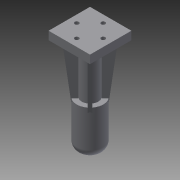
# Autodesk Inventor part: QuadrupedFoot
Saved by Autodesk Inventor 2015 (Build 190159000, 159)
## iProperties
Created: 2015-04-28
Part Number: QuadrupedFoot
Material: ABS Plastic
Document SubType Name: Modeling
Designer: Quinn
Density: 1.06 g/cm^3
Appearance: Smooth - White
Author: Quinn
Autodesk Inventor part; units mm, degrees
ref_plane "YZ Plane" through (0, 0, 0) normal (1, 0, 0) x (0, 1, 0)
ref_plane "XZ Plane" through (0, 0, 0) normal (0, 1, 0) x (-1, 0, 0)
ref_plane "XY Plane" through (0, 0, 0) normal (0, 0, 1) x (1, 0, 0)
sketch "Sketch2" plane through (0, 0, 0) normal (0, 1, 0) x (-1, 0, 0)
  line L0 (3.9404, 4.971) -> (-21.0596, 4.971)
  line L1 (-21.0596, 4.971) -> (-21.0596, -20.029)
  line L2 (-21.0596, -20.029) -> (3.9404, -20.029)
  line L3 (3.9404, -20.029) -> (3.9404, 4.971)
  circle A0 centre (-0.5596, -7.529) radius 1.25
  circle A1 centre (-16.5596, -7.529) radius 1.25
  circle A2 centre (-8.5596, 0.471) radius 1.25
  circle A3 centre (-8.5596, -15.529) radius 1.25
  point P0 (0, 0)
  dimension "d0" = 25
  dimension "d1" = 25
  dimension "d4" = 2.5
  dimension "d5" = 2.5
  dimension "d8" = 2.5
  dimension "d9" = 2.5
  constraints: 8 end point, 4 centre point, 2 parallel, 1 horizontal, 1 perpendicular
  measures "d0" distance of L2.end L1.end
  measures "d1" distance of L1.end L0.end
  measures "d4" diameter of A0
  measures "d5" diameter of A1
  measures "d8" diameter of A2
  measures "d9" diameter of A3
extrude "Extrusion1" add sketch "Sketch2" along normal blind 7
sketch "Sketch3" plane through (0, 0, 0) normal (0, -1, 0) x (1, 0, 0)
  circle A0 centre (8.5596, -15.529) radius 1.25 projected
  circle A1 centre (8.5596, 0.471) radius 1.25 projected
  circle A2 centre (16.5596, -7.529) radius 1.25 projected
  circle A3 centre (0.5596, -7.529) radius 1.25 projected
  line L0 (-3.9404, 4.971) -> (21.0596, 4.971) projected
  line L1 (-3.9404, -20.029) -> (-3.9404, 4.971) projected
  line L2 (21.0596, -20.029) -> (-3.9404, -20.029) projected
  line L3 (21.0596, 4.971) -> (21.0596, -20.029) projected
  circle A4 centre (8.5596, -7.529) radius 5
  point P0 (0, 0)
  dimension "d12" = 10
  constraints: 1 centre point
  measures "d12" diameter of A4
extrude "Extrusion2" add sketch "Sketch3" along normal blind 55 contours A4
sketch "Sketch4" plane through (0, 0, 0) normal (0, -1, 0) x (1, 0, 0)
  circle A0 centre (8.5596, -7.529) radius 5 projected
  circle A1 centre (8.5596, -15.529) radius 1.25 projected
  circle A2 centre (8.5596, 0.471) radius 1.25 projected
  circle A3 centre (16.5596, -7.529) radius 1.25 projected
  circle A4 centre (0.5596, -7.529) radius 1.25 projected
  line L0 (-3.9404, 4.971) -> (21.0596, 4.971) projected
  line L1 (-3.9404, -20.029) -> (-3.9404, 4.971) projected
  line L2 (21.0596, -20.029) -> (-3.9404, -20.029) projected
  line L3 (21.0596, 4.971) -> (21.0596, -20.029) projected
  circle A5 centre (8.5596, -15.529) radius 2.25
  circle A6 centre (16.5596, -7.529) radius 2.25
  circle A7 centre (8.5596, 0.471) radius 2.25
  circle A8 centre (0.5596, -7.529) radius 2.25
  point P0 (0, 0)
  dimension "d15" = 1
  dimension "d16" = 1
  dimension "d17" = 1
  dimension "d18" = 1
  constraints: 4 centre point
  measures "d15" radial gap between concentric circles of A1 A5
  measures "d16" radial gap between concentric circles of A3 A6
  measures "d17" radial gap between concentric circles of A2 A7
  measures "d18" radial gap between concentric circles of A4 A8
extrude "Extrusion3" cut sketch "Sketch4" against normal blind 2 contours A5 | A6 | A7 | A8
ref_plane "Work Plane1" through (-3.9404, 0, -20.029) normal (-0.7071068, 0, 0.7071068) x (0, 1, 0)
sketch "Sketch6" plane through (-3.9404, 0, -20.029) normal (-0.7071068, 0, 0.7071068) x (0, 1, 0)
  line L0 (-55, -12.6777) -> (-55, -22.6777) projected
  line L1 (0, -22.6777) -> (0, -12.6777) projected
  line L2 (0, -12.6777) -> (-55, -12.6777) projected
  line L3 (0, -25.5845) -> (0, -21.0845) projected
  line L4 (0, -14.2708) -> (0, -9.7708) projected
  line L5 (0, -25.5845) -> (0, -21.0845) projected
  line L6 (0, -14.2708) -> (0, -9.7708) projected
  line L7 (0, -22.6777) -> (0, -12.6777) projected
  line L8 (0, -17.6777) -> (0, -35.3553) projected
  line L9 (0, 0) -> (0, -17.6777) projected
  line L10 (0, -17.6777) -> (0, 0) projected
  line L11 (0, -35.3553) -> (0, -17.6777) projected
  line L12 (-55, -12.6777) -> (0, -6.0835)
  line L13 (0, -6.0835) -> (0, -12.6777)
  line L14 (-55, -12.6777) -> (0, -12.6777)
  point P0 (0, -16.9489)
  constraints: 6 end point, 2 collinear, 1 point on line
extrude "Extrusion4" add sketch "Sketch6" along normal mid plane 2
pattern_circular "Circular Pattern1" count 4 over 360 about axis through (8.5596, 0, -7.529) along (0, -1, 0) of "Extrusion4"
sketch "Sketch7" plane through (0, -55, 0) normal (0, -1, 0) x (1, 0, 0)
  arc A0 (5.024, -11.0645) -> (12.0951, -11.0645) centre (8.5596, -7.529) ccw projected
  arc A1 (12.0951, -11.0645) -> (12.0951, -3.9934) centre (8.5596, -7.529) ccw projected
  arc A2 (12.0951, -3.9934) -> (5.024, -3.9934) centre (8.5596, -7.529) ccw projected
  arc A3 (5.024, -3.9934) -> (5.024, -11.0645) centre (8.5596, -7.529) ccw projected
  arc A4 (14.2164, -13.1858) -> (14.2164, -1.8721) centre (8.5596, -7.529) ccw
  arc A5 (2.9027, -13.1858) -> (14.2164, -13.1858) centre (8.5596, -7.529) ccw
  arc A6 (2.9027, -1.8721) -> (2.9027, -13.1858) centre (8.5596, -7.529) ccw
  arc A7 (14.2164, -1.8721) -> (2.9027, -1.8721) centre (8.5596, -7.529) ccw
  point P0 (0, 0)
  dimension "d26" = 3
  constraints: 8 point on circle, 4 centre point, 3 other
  measures "d26" radial gap between concentric circles of A1 A4
extrude "Extrusion5" add sketch "Sketch7" against normal blind 27.4
fillet "Fillet1" radius 5.175 1 edges at (14.2164, -55, -1.8721)
chamfer "Chamfer1" distance 2 angle 45 4 edges at (21.0596, 0, -7.529) (8.5596, 0, -20.029) (-3.9404, 0, -7.529) (8.5596, 0, 4.971)
body "Solid1"
